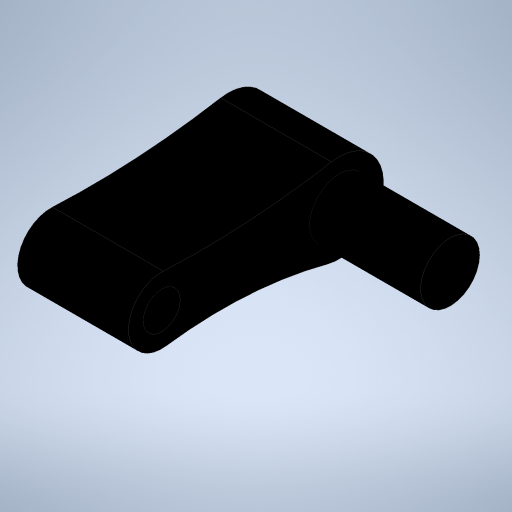
# Autodesk Inventor part: Motoranker
Saved by Autodesk Inventor 2023 (Build 270158000, 158)
## iProperties
Created: 2024-01-25
Part Number: Motoranker
Material: Generisch
Document SubType Name: Modeling
Designer: phili
Density: 1 g/cm^3
Appearance: Vorgabe
Author: phili
Autodesk Inventor part; units mm, degrees
ref_plane "YZ Plane" through (0, 0, 0) normal (1, 0, 0) x (0, 1, 0)
ref_plane "XZ Plane" through (0, 0, 0) normal (0, 1, 0) x (-1, 0, 0)
ref_plane "XY Plane" through (0, 0, 0) normal (0, 0, 1) x (1, 0, 0)
sketch "Skizze1" plane through (0, 0, 0) normal (1, 0, 0) x (0, 1, 0)
  circle A0 centre (0, 9) radius 4.5
  circle A1 centre (0, -15) radius 6
  arc A2 (4.4948, 8.7827) -> (5.9108, -13.9694) centre (107.7663, 3.7901) ccw
  arc A3 (-5.8012, -13.4684) -> (-4.4588, 8.3923) centre (-59.9557, 0.8287) ccw
  circle A4 centre (0, 9) radius 2.5
  point P0 (0, 0)
  dimension "d0" = 9
  dimension "d1" = 12
  dimension "d2" = 15
  dimension "d3" = 9
  dimension "d4" = 0
  dimension "d5" = 0
  dimension "d6" = 5
  constraints: 8 point on circle, 5 centre point, 4 tangent, 1 coincident
  measures "d0" diameter of A0
  measures "d1" diameter of A1
  measures "d2" distance of A1.centre point (0, 0)
  measures "d3" distance of point (0, 0) A0.centre
  measures "d4" horizontal distance of point (0, 0) A0.centre
  measures "d5" horizontal distance of point (0, 0) A1.centre
  measures "d6" diameter of A4
extrude "Extrusion1" add sketch "Skizze1" along normal blind 15
sketch "Skizze2" plane through (15, 0, 0) normal (1, 0, 0) x (0, 0, -1)
  arc A0 (13.4684, -5.8012) -> (13.9694, 5.9108) centre (15, 0) ccw projected
  circle A1 centre (15, 0) radius 4
  point P0 (0, 0)
  dimension "d10" = 8
  constraints: 1 centre point, 1 coincident
  measures "d10" diameter of A1
extrude "Extrusion2" add sketch "Skizze2" along normal blind 15
